Autodesk Inventor part; units mm, degrees
(part 2 of 2)
  dimension "d53" = 14.005
  dimension "d54" = 14.005
  dimension "d55" = 14.005
  dimension "d56" = 14.005
  dimension "d57" = 14.005
  dimension "d58" = 14.005
  dimension "d59" = 14.005
  dimension "d60" = 14.005
  dimension "d61" = 14.005
  dimension "d62" = 14.005
  dimension "d63" = 14.005
  dimension "d64" = 14.005
  constraints: 856 end point, 119 parallel, 117 midpoint, 108 perpendicular, 63 horizontal, 45 point on line, 18 equal length, 11 collinear, 6 coincident, 5 centre point, 4 equal radius, 4 vertical
  measures "d0" distance from line of L55 A243.centre
  measures "d1" distance from line of L52 A243.centre
  measures "d2" distance from line of L54 A270.centre
  measures "d3" distance from line of L53 A270.centre
  measures "d5" distance of L86.end L87.end
  measures "d6" distance of L85.end L86.end
  measures "d7" distance of L92.end L93.end
  measures "d8" distance of L91.end L92.end
  measures "d9" distance of L98.end L99.end
  measures "d10" distance of L97.end L98.end
  measures "d11" distance of L104.end L105.end
  measures "d12" distance of L103.end L104.end
  measures "d13" distance of L110.end L111.end
  measures "d14" distance of L109.end L110.end
  measures "d15" distance of L116.end L117.end
  measures "d16" distance of L115.end L116.end
  measures "d17" distance of L122.end L123.end
  measures "d18" distance of L121.end L122.end
  measures "d19" distance of L128.end L129.end
  measures "d20" distance of L127.end L128.end
  measures "d21" distance of L134.end L135.end
  measures "d22" distance of L133.end L134.end
  measures "d23" distance of L140.end L141.end
  measures "d24" distance of L139.end L140.end
  measures "d25" distance of L146.end L147.end
  measures "d26" distance of L145.end L146.end
  measures "d27" distance of L152.end L153.end
  measures "d28" distance of L151.end L152.end
  measures "d29" distance of L158.end L159.end
  measures "d30" distance of L157.end L158.end
  measures "d31" distance of L164.end L165.end
  measures "d32" distance of L163.end L164.end
  measures "d33" distance of L170.end L171.end
  measures "d34" distance of L169.end L170.end
  measures "d35" distance of L176.end L177.end
  measures "d36" distance of L175.end L176.end
  measures "d37" distance of L182.end L183.end
  measures "d38" distance of L181.end L182.end
  measures "d39" distance of L188.end L189.end
  measures "d40" distance of L187.end L188.end
  measures "d41" distance of L194.end L195.end
  measures "d42" distance of L193.end L194.end
  measures "d43" distance of L200.end L201.end
  measures "d44" distance of L199.end L200.end
  measures "d45" distance of L206.end L207.end
  measures "d46" distance of L205.end L206.end
  measures "d47" distance of L212.end L213.end
  measures "d48" distance of L211.end L212.end
  measures "d49" distance of L218.end L219.end
  measures "d50" distance of L217.end L218.end
  measures "d51" distance of L224.end L225.end
  measures "d52" distance of L223.end L224.end
  measures "d53" distance of L230.end L231.end
  measures "d54" distance of L229.end L230.end
  measures "d55" distance of L236.end L237.end
  measures "d56" distance of L235.end L236.end
  measures "d57" distance of L242.end L243.end
  measures "d58" distance of L241.end L242.end
  measures "d59" distance of L248.end L249.end
  measures "d60" distance of L247.end L248.end
  measures "d61" distance of L254.end L255.end
  measures "d62" distance of L253.end L254.end
  measures "d63" distance of L260.end L261.end
  measures "d64" distance of L259.end L260.end
extrude "Thin base" add sketch "Sketch2" along normal blind 0.5 contours L0 L3 L2 L459 L460 L461 L462 L463 L464 L465 L466 L467 L468 L469 | L5 L6 L7 L447 L446 L445 L444 L443 | L9 L10 L11 L455 L454 L453 L452 L451 | L41 L42 L43 L431 L430 L429 L428 L427 | L45 L46 L47 L439 L438 L437 L436 L435
sketch "Sketch3" plane through (0, 0, 0.5) normal (0, 0, 1) x (1, 0, 0)
  line L0 (265.0048, -148.2602) -> (265.0048, -126.6954)
  line L1 (265.0048, -126.6954) -> (274.6598, -126.6954)
  line L2 (274.6598, -126.6954) -> (274.6598, -107.8454)
  line L3 (274.6598, -107.8454) -> (269.5798, -107.8454)
  line L4 (269.5798, -107.8454) -> (269.5798, -88.7954)
  line L5 (269.5798, -88.7954) -> (260.1818, -88.7954)
  line L6 (260.1818, -88.7954) -> (260.1818, -60.9161)
  line L7 (260.1818, -60.9161) -> (269.4528, -60.9161)
  line L8 (269.4528, -60.9161) -> (269.4528, -40)
  line L9 (269.4528, -40) -> (40, -40)
  line L10 (40, -40) -> (40, -165)
  line L11 (40, -165) -> (272.0064, -165)
  line L12 (272.0064, -165) -> (272.0064, -148.2602)
  line L13 (272.0064, -148.2602) -> (265.0048, -148.2602)
  circle A0 centre (155, -160) radius 3.25
  circle A1 centre (265, -160) radius 3.25
  circle A2 centre (155, -64.8616) radius 3.25
  circle A3 centre (45, -64.8616) radius 3.25
  line L14 (83.7343, -148.3679) -> (97.7393, -148.3679)
  line L15 (97.7393, -148.3679) -> (97.7393, -162.3729)
  line L16 (97.7393, -162.3729) -> (83.7343, -162.3729)
  line L17 (83.7343, -162.3729) -> (83.7343, -148.3679)
  line L18 (59.8583, -148.3679) -> (73.8633, -148.3679)
  line L19 (73.8633, -148.3679) -> (73.8633, -162.3729)
  line L20 (73.8633, -162.3729) -> (59.8583, -162.3729)
  line L21 (59.8583, -162.3729) -> (59.8583, -148.3679)
  line L22 (50.9683, -129.3179) -> (64.9733, -129.3179)
  line L23 (64.9733, -129.3179) -> (64.9733, -143.3229)
  line L24 (64.9733, -143.3229) -> (50.9683, -143.3229)
  line L25 (50.9683, -143.3229) -> (50.9683, -129.3179)
  line L26 (77.1303, -129.3179) -> (91.1353, -129.3179)
  line L27 (91.1353, -129.3179) -> (91.1353, -143.3229)
  line L28 (91.1353, -143.3229) -> (77.1303, -143.3229)
  line L29 (77.1303, -143.3229) -> (77.1303, -129.3179)
  line L30 (96.1803, -129.3179) -> (110.1853, -129.3179)
  line L31 (110.1853, -129.3179) -> (110.1853, -143.3229)
  line L32 (110.1853, -143.3229) -> (96.1803, -143.3229)
  line L33 (96.1803, -143.3229) -> (96.1803, -129.3179)
  line L34 (115.2303, -129.3179) -> (129.2353, -129.3179)
  line L35 (129.2353, -129.3179) -> (129.2353, -143.3229)
  line L36 (129.2353, -143.3229) -> (115.2303, -143.3229)
  line L37 (115.2303, -143.3229) -> (115.2303, -129.3179)
  line L38 (181.3976, -148.3679) -> (195.4026, -148.3679)
  line L39 (195.4026, -148.3679) -> (195.4026, -162.3729)
  line L40 (195.4026, -162.3729) -> (181.3976, -162.3729)
  line L41 (181.3976, -162.3729) -> (181.3976, -148.3679)
  line L42 (134.2803, -129.3179) -> (148.2853, -129.3179)
  line L43 (148.2853, -129.3179) -> (148.2853, -143.3229)
  line L44 (148.2853, -143.3229) -> (134.2803, -143.3229)
  line L45 (134.2803, -143.3229) -> (134.2803, -129.3179)
  line L46 (153.3303, -129.3179) -> (167.3353, -129.3179)
  line L47 (167.3353, -129.3179) -> (167.3353, -143.3229)
  line L48 (167.3353, -143.3229) -> (153.3303, -143.3229)
  line L49 (153.3303, -143.3229) -> (153.3303, -129.3179)
  line L50 (172.3803, -129.3179) -> (186.3853, -129.3179)
  line L51 (186.3853, -129.3179) -> (186.3853, -143.3229)
  line L52 (186.3853, -143.3229) -> (172.3803, -143.3229)
  line L53 (172.3803, -143.3229) -> (172.3803, -129.3179)
  line L54 (191.4303, -129.3179) -> (205.4353, -129.3179)
  line L55 (205.4353, -129.3179) -> (205.4353, -143.3229)
  line L56 (205.4353, -143.3229) -> (191.4303, -143.3229)
  line L57 (191.4303, -143.3229) -> (191.4303, -129.3179)
  line L58 (210.4803, -129.3179) -> (224.4853, -129.3179)
  line L59 (224.4853, -129.3179) -> (224.4853, -143.3229)
  line L60 (224.4853, -143.3229) -> (210.4803, -143.3229)
  line L61 (210.4803, -143.3229) -> (210.4803, -129.3179)
  line L62 (229.5343, -129.3199) -> (243.5393, -129.3199)
  line L63 (243.5393, -129.3199) -> (243.5393, -143.3249)
  line L64 (243.5393, -143.3249) -> (229.5343, -143.3249)
  line L65 (229.5343, -143.3249) -> (229.5343, -129.3199)
  line L66 (248.5743, -129.3399) -> (262.5793, -129.3399)
  line L67 (262.5793, -129.3399) -> (262.5793, -143.3449)
  line L68 (262.5793, -143.3449) -> (248.5743, -143.3449)
  line L69 (248.5743, -143.3449) -> (248.5743, -129.3399)
  line L70 (258.2323, -110.2679) -> (272.2373, -110.2679)
  line L71 (272.2373, -110.2679) -> (272.2373, -124.2729)
  line L72 (272.2373, -124.2729) -> (258.2323, -124.2729)
  line L73 (258.2323, -124.2729) -> (258.2323, -110.2679)
  line L74 (238.9283, -110.2679) -> (252.9333, -110.2679)
  line L75 (252.9333, -110.2679) -> (252.9333, -124.2729)
  line L76 (252.9333, -124.2729) -> (238.9283, -124.2729)
  line L77 (238.9283, -124.2729) -> (238.9283, -110.2679)
  line L78 (219.8783, -110.2679) -> (233.8833, -110.2679)
  line L79 (233.8833, -110.2679) -> (233.8833, -124.2729)
  line L80 (233.8833, -124.2729) -> (219.8783, -124.2729)
  line L81 (219.8783, -124.2729) -> (219.8783, -110.2679)
  line L82 (200.8283, -110.2679) -> (214.8333, -110.2679)
  line L83 (214.8333, -110.2679) -> (214.8333, -124.2729)
  line L84 (214.8333, -124.2729) -> (200.8283, -124.2729)
  line L85 (200.8283, -124.2729) -> (200.8283, -110.2679)
  line L86 (181.7783, -110.2679) -> (195.7833, -110.2679)
  line L87 (195.7833, -110.2679) -> (195.7833, -124.2729)
  line L88 (195.7833, -124.2729) -> (181.7783, -124.2729)
  line L89 (181.7783, -124.2729) -> (181.7783, -110.2679)
  line L90 (162.7283, -110.2679) -> (176.7333, -110.2679)
  line L91 (176.7333, -110.2679) -> (176.7333, -124.2729)
  line L92 (176.7333, -124.2729) -> (162.7283, -124.2729)
  line L93 (162.7283, -124.2729) -> (162.7283, -110.2679)
  line L94 (143.6783, -110.2679) -> (157.6833, -110.2679)
  line L95 (157.6833, -110.2679) -> (157.6833, -124.2729)
  line L96 (157.6833, -124.2729) -> (143.6783, -124.2729)
  line L97 (143.6783, -124.2729) -> (143.6783, -110.2679)
  line L98 (124.6283, -110.2679) -> (138.6333, -110.2679)
  line L99 (138.6333, -110.2679) -> (138.6333, -124.2729)
  line L100 (138.6333, -124.2729) -> (124.6283, -124.2729)
  line L101 (124.6283, -124.2729) -> (124.6283, -110.2679)
  line L102 (105.5783, -110.2679) -> (119.5833, -110.2679)
  line L103 (119.5833, -110.2679) -> (119.5833, -124.2729)
  line L104 (119.5833, -124.2729) -> (105.5783, -124.2729)
  line L105 (105.5783, -124.2729) -> (105.5783, -110.2679)
  line L106 (86.5283, -110.2679) -> (100.5333, -110.2679)
  line L107 (100.5333, -110.2679) -> (100.5333, -124.2729)
  line L108 (100.5333, -124.2729) -> (86.5283, -124.2729)
  line L109 (86.5283, -124.2729) -> (86.5283, -110.2679)
  line L110 (67.4783, -110.2679) -> (81.4833, -110.2679)
  line L111 (81.4833, -110.2679) -> (81.4833, -124.2729)
  line L112 (81.4833, -124.2729) -> (67.4783, -124.2729)
  line L113 (67.4783, -124.2729) -> (67.4783, -110.2679)
  line L114 (81.7023, -91.2179) -> (95.7073, -91.2179)
  line L115 (95.7073, -91.2179) -> (95.7073, -105.2229)
  line L116 (95.7073, -105.2229) -> (81.7023, -105.2229)
  line L117 (81.7023, -105.2229) -> (81.7023, -91.2179)
  line L118 (100.7523, -91.2179) -> (114.7573, -91.2179)
  line L119 (114.7573, -91.2179) -> (114.7573, -105.2229)
  line L120 (114.7573, -105.2229) -> (100.7523, -105.2229)
  line L121 (100.7523, -105.2229) -> (100.7523, -91.2179)
  line L122 (119.8023, -91.2179) -> (133.8073, -91.2179)
  line L123 (133.8073, -91.2179) -> (133.8073, -105.2229)
  line L124 (133.8073, -105.2229) -> (119.8023, -105.2229)
  line L125 (119.8023, -105.2229) -> (119.8023, -91.2179)
  line L126 (138.8523, -91.2179) -> (152.8573, -91.2179)
  line L127 (152.8573, -91.2179) -> (152.8573, -105.2229)
  line L128 (152.8573, -105.2229) -> (138.8523, -105.2229)
  line L129 (138.8523, -105.2229) -> (138.8523, -91.2179)
  line L130 (157.9023, -91.2967) -> (171.9073, -91.2967)
  line L131 (171.9073, -91.2967) -> (171.9073, -105.3017)
  line L132 (171.9073, -105.3017) -> (157.9023, -105.3017)
  line L133 (157.9023, -105.3017) -> (157.9023, -91.2967)
  line L134 (176.9523, -91.2179) -> (190.9573, -91.2179)
  line L135 (190.9573, -91.2179) -> (190.9573, -105.2229)
  line L136 (190.9573, -105.2229) -> (176.9523, -105.2229)
  line L137 (176.9523, -105.2229) -> (176.9523, -91.2179)
  line L138 (196.0023, -91.2179) -> (210.0073, -91.2179)
  line L139 (210.0073, -91.2179) -> (210.0073, -105.2229)
  line L140 (210.0073, -105.2229) -> (196.0023, -105.2229)
  line L141 (196.0023, -105.2229) -> (196.0023, -91.2179)
  line L142 (215.0523, -91.2179) -> (229.0573, -91.2179)
  line L143 (229.0573, -91.2179) -> (229.0573, -105.2229)
  line L144 (229.0573, -105.2229) -> (215.0523, -105.2229)
  line L145 (215.0523, -105.2229) -> (215.0523, -91.2179)
  line L146 (234.1023, -91.2179) -> (248.1073, -91.2179)
  line L147 (248.1073, -91.2179) -> (248.1073, -105.2229)
  line L148 (248.1073, -105.2229) -> (234.1023, -105.2229)
  line L149 (234.1023, -105.2229) -> (234.1023, -91.2179)
  line L150 (253.1523, -91.2179) -> (267.1573, -91.2179)
  line L151 (267.1573, -91.2179) -> (267.1573, -105.2229)
  line L152 (267.1573, -105.2229) -> (253.1523, -105.2229)
  line L153 (253.1523, -105.2229) -> (253.1523, -91.2179)
  line L154 (243.7543, -72.1679) -> (257.7593, -72.1679)
  line L155 (257.7593, -72.1679) -> (257.7593, -86.1729)
  line L156 (257.7593, -86.1729) -> (243.7543, -86.1729)
  line L157 (243.7543, -86.1729) -> (243.7543, -72.1679)
  line L158 (224.7043, -72.1679) -> (238.7093, -72.1679)
  line L159 (238.7093, -72.1679) -> (238.7093, -86.1729)
  line L160 (238.7093, -86.1729) -> (224.7043, -86.1729)
  line L161 (224.7043, -86.1729) -> (224.7043, -72.1679)
  line L162 (205.6543, -72.1679) -> (219.6593, -72.1679)
  line L163 (219.6593, -72.1679) -> (219.6593, -86.1729)
  line L164 (219.6593, -86.1729) -> (205.6543, -86.1729)
  line L165 (205.6543, -86.1729) -> (205.6543, -72.1679)
  line L166 (186.6043, -72.1679) -> (200.6093, -72.1679)
  line L167 (200.6093, -72.1679) -> (200.6093, -86.1729)
  line L168 (200.6093, -86.1729) -> (186.6043, -86.1729)
  line L169 (186.6043, -86.1729) -> (186.6043, -72.1679)
  line L170 (53.2543, -91.2179) -> (67.2593, -91.2179)
  line L171 (67.2593, -91.2179) -> (67.2593, -105.2229)
  line L172 (67.2593, -105.2229) -> (53.2543, -105.2229)
  line L173 (53.2543, -105.2229) -> (53.2543, -91.2179)
  line L174 (167.5543, -72.1679) -> (181.5593, -72.1679)
  line L175 (181.5593, -72.1679) -> (181.5593, -86.1729)
  line L176 (181.5593, -86.1729) -> (167.5543, -86.1729)
  line L177 (167.5543, -86.1729) -> (167.5543, -72.1679)
  line L178 (148.5043, -72.1679) -> (162.5093, -72.1679)
  line L179 (162.5093, -72.1679) -> (162.5093, -86.1729)
  line L180 (162.5093, -86.1729) -> (148.5043, -86.1729)
  line L181 (148.5043, -86.1729) -> (148.5043, -72.1679)
  line L182 (129.4543, -72.1679) -> (143.4593, -72.1679)
  line L183 (143.4593, -72.1679) -> (143.4593, -86.1729)
  line L184 (143.4593, -86.1729) -> (129.4543, -86.1729)
  line L185 (129.4543, -86.1729) -> (129.4543, -72.1679)
  line L186 (110.4043, -72.1679) -> (124.4093, -72.1679)
  line L187 (124.4093, -72.1679) -> (124.4093, -86.1729)
  line L188 (124.4093, -86.1729) -> (110.4043, -86.1729)
  line L189 (110.4043, -86.1729) -> (110.4043, -72.1679)
  line L190 (91.3543, -72.1679) -> (105.3593, -72.1679)
  line L191 (105.3593, -72.1679) -> (105.3593, -86.1729)
  line L192 (105.3593, -86.1729) -> (91.3543, -86.1729)
  line L193 (91.3543, -86.1729) -> (91.3543, -72.1679)
  line L194 (72.3043, -72.1679) -> (86.3093, -72.1679)
  line L195 (86.3093, -72.1679) -> (86.3093, -86.1729)
  line L196 (86.3093, -86.1729) -> (72.3043, -86.1729)
  line L197 (72.3043, -86.1729) -> (72.3043, -72.1679)
  line L198 (48.5263, -72.1679) -> (62.5313, -72.1679)
  line L199 (62.5313, -72.1679) -> (62.5313, -86.1729)
  line L200 (62.5313, -86.1729) -> (48.5263, -86.1729)
  line L201 (48.5263, -86.1729) -> (48.5263, -72.1679)
  line L202 (43.8563, -43.6091) -> (57.8613, -43.6091)
  line L203 (57.8613, -43.6091) -> (57.8613, -57.6141)
  line L204 (57.8613, -57.6141) -> (43.8563, -57.6141)
  line L205 (43.8563, -57.6141) -> (43.8563, -43.6091)
  line L206 (74.9047, -43.3959) -> (88.9097, -43.3959)
  line L207 (88.9097, -43.3959) -> (88.9097, -57.4009)
  line L208 (88.9097, -57.4009) -> (74.9047, -57.4009)
  line L209 (74.9047, -57.4009) -> (74.9047, -43.3959)
  line L210 (98.7203, -43.5111) -> (112.7253, -43.5111)
  line L211 (112.7253, -43.5111) -> (112.7253, -57.5161)
  line L212 (112.7253, -57.5161) -> (98.7203, -57.5161)
  line L213 (98.7203, -57.5161) -> (98.7203, -43.5111)
  line L214 (122.5963, -43.5391) -> (136.6013, -43.5391)
  line L215 (136.6013, -43.5391) -> (136.6013, -57.5441)
  line L216 (136.6013, -57.5441) -> (122.5963, -57.5441)
  line L217 (122.5963, -57.5441) -> (122.5963, -43.5391)
  line L218 (146.4723, -43.5111) -> (160.4773, -43.5111)
  line L219 (160.4773, -43.5111) -> (160.4773, -57.5161)
  line L220 (160.4773, -57.5161) -> (146.4723, -57.5161)
  line L221 (146.4723, -57.5161) -> (146.4723, -43.5111)
  line L222 (170.3483, -43.5111) -> (184.3533, -43.5111)
  line L223 (184.3533, -43.5111) -> (184.3533, -57.5161)
  line L224 (184.3533, -57.5161) -> (170.3483, -57.5161)
  line L225 (170.3483, -57.5161) -> (170.3483, -43.5111)
  line L226 (202.8543, -43.5111) -> (216.8593, -43.5111)
  line L227 (216.8593, -43.5111) -> (216.8593, -57.5161)
  line L228 (216.8593, -57.5161) -> (202.8543, -57.5161)
  line L229 (202.8543, -57.5161) -> (202.8543, -43.5111)
  line L230 (226.7363, -43.5111) -> (240.7413, -43.5111)
  line L231 (240.7413, -43.5111) -> (240.7413, -57.5161)
  line L232 (240.7413, -57.5161) -> (226.7363, -57.5161)
  line L233 (226.7363, -57.5161) -> (226.7363, -43.5111)
  line L234 (250.6123, -43.5111) -> (264.6173, -43.5111)
  line L235 (264.6173, -43.5111) -> (264.6173, -57.5161)
  line L236 (264.6173, -57.5161) -> (250.6123, -57.5161)
  line L237 (250.6123, -57.5161) -> (250.6123, -43.5111)
  line L238 (172.0148, -58.6601) -> (214.7648, -58.6601)
  line L239 (214.7648, -58.6601) -> (214.7648, -65.1601)
  line L240 (214.7648, -65.1601) -> (172.0148, -65.1601)
  line L241 (172.0148, -65.1601) -> (172.0148, -58.6601)
  line L242 (258.1501, -148.6179) -> (258.1501, -161.1179)
  line L243 (258.1501, -161.1179) -> (252.1501, -161.1179)
  line L244 (252.1501, -161.1179) -> (252.1501, -148.6179)
  line L245 (252.1501, -148.6179) -> (254.1501, -148.6179)
  line L246 (254.1501, -148.6179) -> (254.1501, -147.1179)
  line L247 (254.1501, -147.1179) -> (256.1501, -147.1179)
  line L248 (256.1501, -147.1179) -> (256.1501, -148.6179)
  line L249 (256.1501, -148.6179) -> (258.1501, -148.6179)
  line L250 (124.6501, -148.6179) -> (124.6501, -161.1179)
  line L251 (124.6501, -161.1179) -> (118.6501, -161.1179)
  line L252 (118.6501, -161.1179) -> (118.6501, -148.6179)
  line L253 (118.6501, -148.6179) -> (120.6501, -148.6179)
  line L254 (120.6501, -148.6179) -> (120.6501, -147.1179)
  line L255 (120.6501, -147.1179) -> (122.6501, -147.1179)
  line L256 (122.6501, -147.1179) -> (122.6501, -148.6179)
  line L257 (122.6501, -148.6179) -> (124.6501, -148.6179)
  line L258 (75.2568, -91.4679) -> (75.2568, -103.9679)
  line L259 (75.2568, -103.9679) -> (69.2568, -103.9679)
  line L260 (69.2568, -103.9679) -> (69.2568, -91.4679)
  line L261 (69.2568, -91.4679) -> (71.2568, -91.4679)
  line L262 (71.2568, -91.4679) -> (71.2568, -89.9679)
  line L263 (71.2568, -89.9679) -> (73.2568, -89.9679)
  line L264 (73.2568, -89.9679) -> (73.2568, -91.4679)
  line L265 (73.2568, -91.4679) -> (75.2568, -91.4679)
  line L266 (51.2568, -91.4679) -> (51.2568, -103.9679)
  line L267 (51.2568, -103.9679) -> (45.2568, -103.9679)
  line L268 (45.2568, -103.9679) -> (45.2568, -91.4679)
  line L269 (45.2568, -91.4679) -> (47.2568, -91.4679)
  line L270 (47.2568, -91.4679) -> (47.2568, -89.9679)
  line L271 (47.2568, -89.9679) -> (49.2568, -89.9679)
  line L272 (49.2568, -89.9679) -> (49.2568, -91.4679)
  line L273 (49.2568, -91.4679) -> (51.2568, -91.4679)
  line L274 (60.1473, -110.2679) -> (60.1473, -124.2729)
  line L275 (60.1473, -124.2729) -> (46.7679, -124.2729)
  arc A4 (46.1423, -123.9574) -> (46.7679, -124.2729) centre (45, -127) ccw
  line L276 (46.1423, -123.9574) -> (46.1423, -110.2679)
  line L277 (46.1423, -110.2679) -> (60.1473, -110.2679)
  circle A5 centre (50.8588, -50.6116) radius 2.55 construction
  line L278 (41.3588, -41.1116) -> (60.3588, -41.1116)
  line L279 (60.3588, -41.1116) -> (60.3588, -60.1116)
  line L280 (60.3588, -60.1116) -> (41.3588, -60.1116)
  line L281 (41.3588, -60.1116) -> (41.3588, -41.1116)
  line L282 (41.3588, -41.1116) -> (60.3588, -60.1116) construction
  line L283 (60.3588, -41.1116) -> (41.3588, -60.1116) construction
  line L284 (72.4072, -41.1116) -> (186.8508, -41.1116)
  line L285 (186.8508, -41.1116) -> (186.8508, -58.6601)
  line L286 (172.0148, -60.1116) -> (72.4072, -60.1116)
  line L287 (72.4072, -60.1116) -> (72.4072, -41.1116)
  line L288 (200.3568, -41.1116) -> (269.4528, -41.1116)
  line L289 (269.4528, -41.1116) -> (269.4528, -60.1116)
  line L290 (269.4528, -60.1116) -> (214.7648, -60.1116)
  line L291 (200.3568, -58.6601) -> (200.3568, -41.1116)
  line L292 (41.3588, -69.6704) -> (260.1818, -69.6704)
  line L293 (41.3588, -69.6704) -> (41.3588, -146)
  line L294 (41.3588, -146) -> (55.3588, -146)
  line L295 (55.3588, -146) -> (55.3588, -164.8704)
  line L296 (55.3588, -164.8704) -> (272.0064, -164.8704)
  line L297 (172.0148, -60.1116) -> (172.0148, -58.6601)
  line L298 (172.0148, -58.6601) -> (186.8508, -58.6601)
  line L299 (172.0148, -58.6601) -> (214.7648, -58.6601)
  line L300 (200.3568, -58.6601) -> (214.7648, -58.6601)
  line L301 (214.7648, -58.6601) -> (214.7648, -60.1116)
  circle A6 centre (81.9072, -50.3984) radius 2.55 construction
  circle A7 centre (177.3508, -50.5136) radius 2.55 construction
  circle A8 centre (209.8568, -50.5136) radius 2.55 construction
  circle A9 centre (55.5288, -79.1704) radius 2.55 construction
  circle A10 centre (66.8608, -155.3704) radius 2.55 construction
  point P0 (0, 0)
extrude "Switch platforms" add sketch "Sketch3" along normal blind 2.5 contours L13 L12 L296 L295 L294 L293 L292 L6 L5 L4 L3 L2 L1 L0 | L8 L290 L239 L238 L291 L288 | L238 L241 L286 L287 L284 L285 | L278 L279 L280 L281
sketch "Sketch4" plane through (0, 0, 0) normal (0, 0, -1) x (-1, 0, 0)
  line L0 (-75.2568, -105.2179) -> (-69.2568, -105.2179)
  line L1 (-75.2568, -103.9679) -> (-69.2568, -103.9679) projected
  line L2 (-69.2568, -105.2179) -> (-69.2568, -94.7179)
  line L3 (-69.2568, -94.7179) -> (-51.2568, -94.7179)
  line L4 (-51.2568, -91.4679) -> (-51.2568, -103.9679) projected
  line L5 (-51.2568, -94.7179) -> (-51.2568, -105.2179)
  line L6 (-51.2568, -105.2179) -> (-45.2568, -105.2179)
  line L7 (-45.2568, -103.9679) -> (-45.2568, -91.4679) projected
  line L8 (-45.2568, -105.2179) -> (-45.2568, -88.2179)
  line L9 (-45.2568, -88.2179) -> (-75.2568, -88.2179)
  line L10 (-75.2568, -88.2179) -> (-75.2568, -105.2179)
  line L11 (-53.2543, -91.2179) -> (-67.2593, -91.2179) projected
  line L12 (-75.2568, -91.4679) -> (-75.2568, -103.9679) projected
  line L13 (-69.2568, -103.9679) -> (-69.2568, -91.4679) projected
  line L14 (-258.1501, -162.3679) -> (-258.1501, -145.3679)
  line L15 (-258.1501, -148.6179) -> (-258.1501, -161.1179) projected
  line L16 (-258.1501, -145.3679) -> (-118.6501, -145.3679)
  line L17 (-118.6501, -145.3679) -> (-118.6501, -162.3679)
  line L18 (-118.6501, -161.1179) -> (-118.6501, -148.6179) projected
  line L19 (-118.6501, -162.3679) -> (-124.6501, -162.3679)
  line L20 (-124.6501, -162.3679) -> (-124.6501, -151.8679)
  line L21 (-124.6501, -148.6179) -> (-124.6501, -161.1179) projected
  line L22 (-124.6501, -151.8679) -> (-252.1501, -151.8679)
  line L23 (-252.1501, -161.1179) -> (-252.1501, -148.6179) projected
  line L24 (-252.1501, -151.8679) -> (-252.1501, -162.3679)
  line L25 (-252.1501, -162.3679) -> (-258.1501, -162.3679)
  line L26 (-181.3976, -148.3679) -> (-195.4026, -148.3679) projected
  point P0 (0, 0)
  dimension "d155" = 3.5
  dimension "d156" = 3
  dimension "d157" = 17
  dimension "d158" = 3.5
  dimension "d159" = 3
  dimension "d160" = 17
  constraints: 32 end point, 11 perpendicular, 8 collinear, 6 point on line, 1 parallel
  measures "d155" distance between parallel lines of L3 L11
  measures "d156" distance between parallel lines of L9 L11
  measures "d157" distance between parallel lines of L0 L9
  measures "d158" distance between parallel lines of L22 L26
  measures "d159" distance between parallel lines of L16 L26
  measures "d160" distance between parallel lines of L25 L16
extrude "Stabilizer cuts" cut sketch "Sketch4" against normal blind 2
sketch "Sketch5" plane through (269.4528, -60.9161, 0) normal (1, 0, 0) x (0, 0, -1)
  line L0 (0, 0) -> (0, 20.9161) projected
  line L1 (-0.5, 19.8045) -> (-3, 19.8045) projected
  line L2 (0, 0.8045) -> (-1.5, 0.8045)
  line L3 (-1.5, 0.8045) -> (-1.5, 19.8045)
  line L4 (-1.5, 19.8045) -> (0, 19.8045)
  line L5 (0, 19.8045) -> (0, 0.8045)
  line L6 (-0.5, 0.8045) -> (-3, 0.8045) projected
  point P0 (0, 60.9161)
  dimension "d163" = 1.5
  constraints: 8 end point, 2 parallel, 2 point on line, 1 collinear, 1 horizontal, 1 perpendicular
  measures "d163" distance of L3.end L4.end
extrude "underlap 1" cut sketch "Sketch5" against normal blind 2
sketch "Sketch6" plane through (269.5798, -107.8454, 0) normal (1, 0, 0) x (0, 0, -1)
  line L0 (0, 19.05) -> (-3, 19.05) projected
  line L1 (0, 0) -> (-1.5, 0)
  line L2 (-1.5, 0) -> (-1.5, 19.05)
  line L3 (-1.5, 19.05) -> (0, 19.05)
  line L4 (0, 19.05) -> (0, 0)
  point P0 (0, 107.8454)
  constraints: 8 end point, 2 parallel, 1 horizontal, 1 midpoint, 1 perpendicular
extrude "underlap 3" cut sketch "Sketch6" against normal blind 2
sketch "Sketch7" plane through (265.0048, -148.2602, 0) normal (1, 0, 0) x (0, 0, -1)
  line L0 (0, 21.5648) -> (-3, 21.5648) projected
  line L1 (0, 0) -> (-1.5, 0)
  line L2 (-1.5, 0) -> (-1.5, 21.5648)
  line L3 (-1.5, 21.5648) -> (0, 21.5648)
  line L4 (0, 21.5648) -> (0, 0)
  point P0 (0, 148.2602)
  constraints: 8 end point, 2 parallel, 1 horizontal, 1 midpoint, 1 perpendicular
extrude "underlap 5" cut sketch "Sketch7" against normal blind 2
sketch "Sketch8" plane through (272.0064, -165, 0) normal (1, 0, 0) x (0, 0, -1)
  line L0 (0, 16.7398) -> (-3, 16.7398) projected
  line L1 (-3, 0.1296) -> (-1.4, 0.1296)
  line L2 (-1.4, 0.1296) -> (-1.4, 16.7398)
  line L3 (-1.4, 16.7398) -> (-3, 16.7398)
  line L4 (-3, 16.7398) -> (-3, 0.1296)
  point P0 (0, 165)
  dimension "d170" = 1.6
  constraints: 8 end point, 2 parallel, 1 horizontal, 1 perpendicular, 1 point on line
  measures "d170" distance of L3.end L2.end
extrude "underlap 6" cut sketch "Sketch8" against normal blind 2
sketch "Sketch9" plane through (274.6598, -126.6954, 0) normal (1, 0, 0) x (0, 0, -1)
  line L0 (0, 18.85) -> (-3, 18.85) projected
  line L1 (-3, 0) -> (-1.4, 0)
  line L2 (-1.4, 0) -> (-1.4, 18.85)
  line L3 (-1.4, 18.85) -> (-3, 18.85)
  line L4 (-3, 18.85) -> (-3, 0)
  point P0 (0, 126.6954)
  dimension "d173" = 1.6
  constraints: 8 end point, 2 parallel, 1 horizontal, 1 perpendicular, 1 point on line
  measures "d173" distance of L3.end L2.end
extrude "underlap 4" cut sketch "Sketch9" against normal blind 2
sketch "Sketch10" plane through (260.1818, -88.7954, 0) normal (1, 0, 0) x (0, 0, -1)
  line L0 (-3, 0) -> (-3, 19.125) projected
  line L1 (0, 0) -> (-3, 0) projected
  line L2 (-3, 19.125) -> (-1.4, 19.125)
  line L3 (-1.4, 19.125) -> (-1.4, 0)
  line L4 (-1.4, 0) -> (-3, 0)
  line L5 (-3, 0) -> (-3, 19.125)
  point P0 (0, 88.7954)
  dimension "d176" = 1.6
  constraints: 8 end point, 2 parallel, 1 horizontal, 1 perpendicular, 1 point on line
  measures "d176" distance of L3.end L4.end
extrude "underlap 2" cut sketch "Sketch10" against normal blind 2
sketch "Sketch11" plane through (0, 0, 3) normal (0, 0, 1) x (1, 0, 0)
  line L0 (215.7004, -152.4909) -> (226.9992, -152.4909) construction
  line L1 (226.9992, -152.4909) -> (226.9992, -157.5573) construction
  line L2 (226.9992, -157.5573) -> (215.7004, -157.5573) construction
  line L3 (215.7004, -157.5573) -> (215.7004, -152.4909) construction
  line L4 (220.9701, -152.4909) -> (218.6548, -157.5573)
  line L5 (218.6548, -157.5573) -> (218.1153, -157.5573)
  line L6 (218.1153, -157.5573) -> (215.7004, -152.4909)
  line L7 (215.7004, -152.4909) -> (217.0573, -152.4909)
  line L8 (217.0573, -152.4909) -> (218.3768, -155.3457)
  line L9 (218.3768, -155.3457) -> (219.6299, -152.4909)
  line L10 (219.6299, -152.4909) -> (220.9701, -152.4909)
  line L11 (222.8166, -152.4909) -> (222.8166, -157.4909)
  line L12 (222.8166, -157.4909) -> (221.5718, -157.4909)
  line L13 (221.5718, -157.4909) -> (221.5718, -152.4909)
  line L14 (221.5718, -152.4909) -> (222.8166, -152.4909)
  point P0 (0, 0)
  constraints: 2 other
extrude "Extrusion10" cut sketch "Sketch11" against normal blind 0.5
sketch "Sketch12" plane through (0, 0, 0.5) normal (0, 0, 1) x (1, 0, 0)
  line L0 (72.4072, -60.1116) -> (172.0148, -60.1116) projected
  line L1 (172.0148, -60.1116) -> (186.8508, -60.1116)
  line L2 (186.8508, -58.6601) -> (200.3568, -58.6601) projected
  line L3 (186.8508, -60.1116) -> (186.8508, -58.6601)
  line L4 (186.8508, -58.6601) -> (200.3568, -58.6601)
  line L5 (214.7648, -65.1601) -> (172.0148, -65.1601) projected
  line L6 (200.3568, -58.6601) -> (200.3568, -60.1116)
  line L7 (200.3568, -60.1116) -> (214.7648, -60.1116)
  line L8 (214.7648, -58.6601) -> (214.7648, -65.1601) projected
  line L9 (200.3568, -41.1116) -> (200.3568, -58.6601) projected
  line L10 (172.0148, -65.1601) -> (172.0148, -60.1116) projected
  line L11 (214.7648, -65.1601) -> (172.0148, -65.1601) projected
  line L12 (214.7648, -60.1116) -> (214.7648, -65.1601) projected
  point P0 (0, 0)
  constraints: 10 end point, 3 point on line, 2 perpendicular, 1 collinear, 1 horizontal, 1 parallel
ref_plane "Work Plane1" through (39.9992, -165.0028, 0) normal (0, 0, 1) x (1, 0, 0)
extrude "Extrusion11" add sketch "Sketch12" against normal up to surface (0.5 mm away)
sketch "Sketch13" plane through (0, 0, 0.5) normal (0, 0, 1) x (1, 0, 0)
  line L0 (172.0148, -58.6601) -> (186.8508, -58.6601) projected
  line L1 (172.0148, -60.1116) -> (172.0148, -58.6601) projected
  line L2 (186.8508, -60.1116) -> (172.0148, -60.1116) projected
  line L3 (186.8508, -58.6601) -> (186.8508, -60.1116) projected
  line L4 (200.3568, -58.6601) -> (214.7648, -58.6601) projected
  line L5 (200.3568, -60.1116) -> (200.3568, -58.6601) projected
  line L6 (214.7648, -58.6601) -> (214.7648, -60.1116) projected
  line L7 (214.7648, -60.1116) -> (200.3568, -60.1116) projected
  point P0 (0, 0)
ref_plane "Work Plane2" through (39.9992, -165.0028, 0) normal (0, 0, 1) x (1, 0, 0)
extrude "Extrusion12" add sketch "Sketch13" against normal up to surface (0.5 mm away)
sketch "Sketch14" plane through (0, 0, 0.5) normal (0, 0, 1) x (1, 0, 0)
  line L0 (172.0148, -60.1116) -> (172.0148, -58.6601) projected
  line L1 (172.0148, -58.6601) -> (186.8508, -58.6601) projected
  line L2 (186.8508, -60.1116) -> (172.0148, -60.1116) projected
  line L3 (186.8508, -58.6601) -> (186.8508, -60.1116) projected
  line L4 (200.3568, -60.1116) -> (200.3568, -58.6601) projected
  line L5 (200.3568, -58.6601) -> (214.7648, -58.6601) projected
  line L6 (214.7648, -58.6601) -> (214.7648, -60.1116) projected
  line L7 (214.7648, -60.1116) -> (200.3568, -60.1116) projected
  point P0 (0, 0)
extrude "Fill in raised F5/6 platform" add sketch "Sketch13" along normal up to surface (2.5 mm away)
equation "\"d5\" = sw"
equation "\"d6\" = sw"
equation "\"d7\" = sw"
equation "\"d8\" = sw"
equation "\"d9\" = sw"
equation "\"d10\" = sw"
equation "\"d11\" = sw"
equation "\"d12\" = sw"
equation "\"d13\" = sw"
equation "\"d14\" = sw"
equation "\"d15\" = sw"
equation "\"d16\" = sw"
equation "\"d17\" = sw"
equation "\"d18\" = sw"
equation "\"d19\" = sw"
equation "\"d20\" = sw"
equation "\"d21\" = sw"
equation "\"d22\" = sw"
equation "\"d23\" = sw"
equation "\"d24\" = sw"
equation "\"d25\" = sw"
equation "\"d26\" = sw"
equation "\"d27\" = sw"
equation "\"d28\" = sw"
equation "\"d29\" = sw"
equation "\"d30\" = sw"
equation "\"d31\" = sw"
equation "\"d32\" = sw"
equation "\"d33\" = sw"
equation "\"d34\" = sw"
equation "\"d35\" = sw"
equation "\"d36\" = sw"
equation "\"d37\" = sw"
equation "\"d38\" = sw"
equation "\"d39\" = sw"
equation "\"d40\" = sw"
equation "\"d41\" = sw"
equation "\"d42\" = sw"
equation "\"d43\" = sw"
equation "\"d44\" = sw"
equation "\"d45\" = sw"
equation "\"d46\" = sw"
equation "\"d47\" = sw"
equation "\"d48\" = sw"
equation "\"d49\" = sw"
equation "\"d50\" = sw"
equation "\"d51\" = sw"
equation "\"d52\" = sw"
equation "\"d53\" = sw"
equation "\"d54\" = sw"
equation "\"d55\" = sw"
equation "\"d56\" = sw"
equation "\"d57\" = sw"
equation "\"d58\" = sw"
equation "\"d59\" = sw"
equation "\"d60\" = sw"
equation "\"d61\" = sw"
equation "\"d62\" = sw"
equation "\"d63\" = sw"
equation "\"d64\" = sw"
equation "\"sw\" = 14.005"
equation "\"d65\" = sw"
equation "\"d66\" = sw"
equation "\"d67\" = sw"
equation "\"d68\" = sw"
equation "\"d69\" = sw"
equation "\"d70\" = sw"
equation "\"d71\" = sw"
equation "\"d72\" = sw"
equation "\"d73\" = sw"
equation "\"d74\" = sw"
equation "\"d75\" = sw"
equation "\"d76\" = sw"
equation "\"d77\" = sw"
equation "\"d78\" = sw"
equation "\"d79\" = sw"
equation "\"d80\" = sw"
equation "\"d81\" = sw"
equation "\"d82\" = sw"
equation "\"d83\" = sw"
equation "\"d84\" = sw"
equation "\"d85\" = sw"
equation "\"d86\" = sw"
equation "\"d87\" = sw"
equation "\"d88\" = sw"
equation "\"d89\" = sw"
equation "\"d90\" = sw"
equation "\"d91\" = sw"
equation "\"d92\" = sw"
equation "\"d93\" = sw"
equation "\"d94\" = sw"
equation "\"d95\" = sw"
equation "\"d96\" = sw"
equation "\"d97\" = sw"
equation "\"d98\" = sw"
equation "\"d99\" = sw"
equation "\"d100\" = sw"
equation "\"d101\" = sw"
equation "\"d102\" = sw"
equation "\"d103\" = sw"
equation "\"d104\" = sw"
equation "\"d105\" = sw"
equation "\"d106\" = sw"
equation "\"d107\" = sw"
equation "\"d108\" = sw"
equation "\"d109\" = sw"
equation "\"d110\" = sw"
equation "\"d111\" = sw"
equation "\"d112\" = sw"
equation "\"d113\" = sw"
equation "\"d114\" = sw"
equation "\"d115\" = sw"
equation "\"d116\" = sw"
equation "\"d117\" = sw"
equation "\"d118\" = sw"
body "Solid1"
